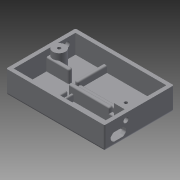
# Autodesk Inventor part: box
Saved by Autodesk Inventor 2014 SP2 (Build 180246200, 246)
## iProperties
Created: 2024-05-21
Part Number: box
Material: Generic
Document SubType Name: Sheet Metal
Designer: GauchoHP
Density: 1 g/cm^3
Sheet Metal Rule: Default_mm
Appearance: Default
Author: GauchoHP
Autodesk Inventor part; units mm, degrees
ref_plane "YZ Plane" through (0, 0, 0) normal (1, 0, 0) x (0, 1, 0)
ref_plane "XZ Plane" through (0, 0, 0) normal (0, 1, 0) x (-1, 0, 0)
ref_plane "XY Plane" through (0, 0, 0) normal (0, 0, 1) x (1, 0, 0)
sketch "Sketch1" plane through (0, 0, 0) normal (0, 0, 1) x (1, 0, 0)
  line L0 (-39, 17.5) -> (39, 17.5)
  line L1 (39, 17.5) -> (39, -37.5)
  line L2 (39, -37.5) -> (-39, -37.5)
  line L3 (-39, -37.5) -> (-39, 17.5)
  point P0 (0, 0)
  dimension "d0" = 78
  dimension "d1" = 55
  dimension "d2" = 17.5
  dimension "d3" = 39
  constraints: 8 end point, 2 parallel, 1 horizontal, 1 perpendicular
  measures "d0" distance of L0.start L0.end
  measures "d1" distance of L2.end L0.start
  measures "d2" distance from line of point (0, 0) L0
  measures "d3" distance from line of point (0, 0) L3
extrude "Extrusion1" add sketch "Sketch1" along normal blind 3
sketch "Sketch2" plane through (0, 0, 3) normal (0, 0, 1) x (1, 0, 0)
  line L0 (39, 17.5) -> (-39, 17.5) projected
  line L1 (-39, 17.5) -> (-39, -37.5) projected
  line L2 (-39, -37.5) -> (39, -37.5) projected
  line L3 (39, -37.5) -> (39, 17.5) projected
  line L4 (-36, 14.5) -> (36, 14.5)
  line L5 (36, 14.5) -> (36, -34.5)
  line L6 (36, -34.5) -> (-36, -34.5)
  line L7 (-36, -34.5) -> (-36, 14.5)
  point P0 (0, 0)
  dimension "d6" = 3
  constraints: 8 end point, 3 other
  measures "d6" distance between parallel lines of L1 L7
extrude "Extrusion2" add sketch "Sketch2" along normal blind 15
sketch "Sketch3" plane through (0, 0, 3) normal (0, 0, 1) x (1, 0, 0)
  line L0 (36, -34.5) -> (36, 14.5) projected
  line L1 (-36, -34.5) -> (36, -34.5) projected
  line L2 (36, -18.5) -> (-7.5, -18.5)
  line L3 (-9, -17) -> (-9, -17)
  line L4 (-7.5, -15.5) -> (36, -15.5)
  line L5 (36, -15.5) -> (36, -18.5)
  line L6 (-36, 14.5) -> (-36, -34.5) projected
  line L7 (-36, -5.5) -> (-19.5, -5.5)
  line L8 (-18, -7) -> (-18, -7)
  line L9 (-19.5, -8.5) -> (-36, -8.5)
  line L10 (-36, -8.5) -> (-36, -5.5)
  arc A0 (-19.5, -8.5) -> (-18, -7) centre (-19.5, -7) ccw
  arc A1 (-18, -7) -> (-19.5, -5.5) centre (-19.5, -7) ccw
  arc A2 (-7.5, -15.5) -> (-9, -17) centre (-7.5, -17) ccw
  arc A3 (-9, -17) -> (-7.5, -18.5) centre (-7.5, -17) ccw
  point P0 (0, 0)
  point P1 (-9, -15.5)
  point P2 (-9, -18.5)
  point P3 (-18, -8.5)
  point P4 (-18, -5.5)
  dimension "d9" = 3
  dimension "d10" = 45
  dimension "d11" = 16
  dimension "d17" = 18
  dimension "d18" = 3
  dimension "d19" = 26
  dimension "d57" = 1.5
  constraints: 16 end point, 10 point on line, 8 point on circle, 8 tangent, 4 centre point, 4 parallel, 3 equal radius, 2 horizontal, 2 perpendicular
  measures "d9" distance of point (-9, -18.5) point (-9, -15.5)
  measures "d10" distance of point (-9, -15.5) L4.end
  measures "d11" distance between parallel lines of L1 L2
  measures "d17" distance of point (-18, -8.5) L9.end
  measures "d18" distance of point (-18, -5.5) point (-18, -8.5)
  measures "d19" distance between parallel lines of L1 L9
  measures "d57" radius of A0
extrude "Extrusion3" add sketch "Sketch3" along normal blind 10
sketch "Sketch4" plane through (0, 0, 13) normal (0, 0, 1) x (1, 0, 0)
  line L0 (36, -15.5) -> (-7.5, -15.5) projected
  line L1 (-7.5, -18.5) -> (36, -18.5) projected
  line L2 (23.9349, -15.5) -> (26.9349, -15.5)
  line L3 (26.9349, -15.5) -> (26.9349, -18.5)
  line L4 (26.9349, -18.5) -> (23.9349, -18.5)
  line L5 (23.9349, -18.5) -> (23.9349, -15.5)
  point P0 (-9, -15.5)
  point P1 (-9, -18.5)
  point P2 (0, 0)
  dimension "d14" = 3
  constraints: 8 end point, 2 parallel, 2 point on line, 1 horizontal, 1 perpendicular
  measures "d14" distance of L2.start L2.end
extrude "Extrusion4" cut sketch "Sketch4" against normal blind 4
sketch "Sketch5" plane through (36, -34.5, 18) normal (-1, 0, 0) x (0, 0, 1)
  circle A0 centre (-5, 14) radius 2
  line L0 (-15, 0) -> (0, 0) projected
  line L1 (-15, 0) -> (-15, 16) projected
  line L2 (-15, 2) -> (-8.5, 2)
  line L3 (-8.5, 2) -> (-8.5, 14)
  line L4 (-8.5, 14) -> (-15, 14)
  line L5 (-15, 14) -> (-15, 2)
  line L6 (0, 49) -> (0, 0) projected
  line L7 (-5, 16) -> (-15, 16) projected
  point P0 (-18, 34.5)
  dimension "d20" = 4
  dimension "d38" = 14
  dimension "d39" = 12
  dimension "d40" = 2
  dimension "d41" = 6.5
  dimension "d42" = 0
  dimension "d62" = 5
  dimension "d94" = 16
  constraints: 8 end point, 2 parallel, 1 centre point, 1 horizontal, 1 perpendicular
  measures "d20" diameter of A0
  measures "d38" distance from line of L0 A0.centre
  measures "d39" distance of L2.end L3.end
  measures "d40" distance between parallel lines of L0 L2
  measures "d41" distance of L3.end L4.end
  measures "d42" distance between parallel lines of L1 L5
  measures "d62" distance from line of L6 A0.centre
  measures "d94" distance between parallel lines of L0 L7
extrude "Extrusion5" cut sketch "Sketch5" against normal blind 4
sketch "Sketch6" plane through (0, 0, 3) normal (0, 0, 1) x (1, 0, 0)
  line L0 (36, 14.5) -> (-36, 14.5) projected
  line L1 (-14, 14.5) -> (-11, 14.5)
  line L2 (-11, 14.5) -> (-11, -7)
  line L3 (-12.5, -8.5) -> (-12.5, -8.5)
  line L4 (-14, -7) -> (-14, 14.5)
  line L5 (36, -15.5) -> (36, 14.5) projected
  line L6 (-7.5, -15.5) -> (36, -15.5) projected
  line L7 (24.5, -11.5) -> (-7.5, -11.5)
  line L8 (-9, -10) -> (-9, -10)
  line L9 (-7.5, -8.5) -> (24.5, -8.5)
  line L10 (26, -10) -> (26, -10)
  arc A0 (26, -10) -> (24.5, -8.5) centre (24.5, -10) ccw
  arc A1 (24.5, -11.5) -> (26, -10) centre (24.5, -10) ccw
  arc A2 (-9, -10) -> (-7.5, -11.5) centre (-7.5, -10) ccw
  arc A3 (-7.5, -8.5) -> (-9, -10) centre (-7.5, -10) ccw
  arc A4 (-12.5, -8.5) -> (-11, -7) centre (-12.5, -7) ccw
  arc A5 (-14, -7) -> (-12.5, -8.5) centre (-12.5, -7) ccw
  point P0 (0, 0)
  point P1 (-11, -8.5)
  point P2 (-14, -8.5)
  point P3 (-9, -15.5)
  point P4 (26, -11.5)
  point P5 (-9, -8.5)
  point P6 (-9, -11.5)
  point P7 (26, -8.5)
  dimension "d23" = 3
  dimension "d24" = 23
  dimension "d25" = 0
  dimension "d33" = 47
  dimension "d35" = 3
  dimension "d36" = 4
  dimension "d37" = 23
  dimension "d54" = 35
  dimension "d55" = 10
  dimension "d56" = 1.5
  constraints: 16 end point, 12 point on circle, 12 point on line, 12 tangent, 6 centre point, 5 equal radius, 4 parallel, 2 horizontal, 2 perpendicular
  measures "d23" distance of point (-11, -8.5) point (-14, -8.5)
  measures "d24" distance of L1.end point (-11, -8.5)
  measures "d25" distance between parallel lines of L0 L1
  measures "d33" distance between parallel lines of L2 L5
  measures "d35" distance of point (-9, -11.5) point (-9, -8.5)
  measures "d36" distance between parallel lines of L7 L6
  measures "d37" distance between parallel lines of L0 L9
  measures "d54" distance between parallel lines of L10 L8
  measures "d55" distance between parallel lines of L5 L10
  measures "d56" radius of A0
extrude "Extrusion6" add sketch "Sketch6" along normal blind 5
chamfer "Chamfer1" distance 2 angle 45 4 edges at (37.5, -20.5, 3) (37.5, -32.5, 3) (37.5, -32.5, 9.5) (37.5, -20.5, 9.5)
sketch "Sketch8" plane through (0, 0, 3) normal (0, 0, 1) x (1, 0, 0)
  circle A0 centre (32, -13.5) radius 5
  line L0 (39, 17.5) -> (39, -37.5) projected
  circle A1 centre (32, -13.5) radius 1.25
  line L1 (36, -34.5) -> (36, 14.5) projected
  line L2 (-36, 14.5) -> (-36, -5.5) projected
  line L3 (-36, -5.5) -> (-19.5, -5.5) projected
  circle A2 centre (-32, -2.5) radius 5
  line L4 (-39, -37.5) -> (-39, 17.5) projected
  line L5 (39, 17.5) -> (-39, 17.5) projected
  circle A3 centre (-32, -2.5) radius 1.25
  point P0 (0, 0)
  point P1 (36, -8.5)
  dimension "d46" = 10
  dimension "d47" = 7
  dimension "d50" = 2.5
  dimension "d51" = 4
  dimension "d63" = 10
  dimension "d64" = 3
  dimension "d65" = 4
  dimension "d66" = 7
  dimension "d67" = 20
  dimension "d68" = 31
  dimension "d69" = 2.5
  constraints: 4 centre point, 2 coincident
  measures "d46" diameter of A0
  measures "d47" distance from line of L0 A0.centre
  measures "d50" diameter of A1
  measures "d51" distance from line of L1 A1.centre
  measures "d63" diameter of A2
  measures "d64" distance from line of L3 A2.centre
  measures "d65" distance from line of L2 A2.centre
  measures "d66" distance from line of L4 A2.centre
  measures "d67" distance from line of A2.centre L5
  measures "d68" distance from line of L5 A0.centre
  measures "d69" diameter of A3
extrude "Extrusion7" add sketch "Sketch8" along normal blind 15
sketch "Sketch10" plane through (-36, -34.5, 18) normal (1, 0, 0) x (0, 0, -1)
  circle A0 centre (5, 42) radius 2.5
  line L0 (0, 0) -> (0, 49) projected
  line L1 (15, 49) -> (0, 49) projected
  point P0 (18, 34.5)
  dimension "d58" = 5
  dimension "d61" = 5
  dimension "d71" = 7
  constraints: 1 centre point
  measures "d58" diameter of A0
  measures "d61" distance from line of L0 A0.centre
  measures "d71" distance from line of L1 A0.centre
extrude "Extrusion9" cut sketch "Sketch10" against normal blind 3
fillet "Fillet1" radius 1 4 edges at (39, -37.5, 9) (39, 17.5, 9) (-39, 17.5, 9) (-39, -37.5, 9)
sketch "Sketch11" plane through (0, 0, 13) normal (0, 0, 1) x (1, 0, 0)
  arc A0 (32, -18.5) -> (36, -16.5) centre (32, -13.5) ccw projected
  line L0 (32, -18.5) -> (36, -18.5) projected
  line L1 (36, -16.5) -> (36, -18.5) projected
  point P0 (0, 0)
extrude "Extrusion10" add sketch "Sketch11" along normal blind 5
sketch "Sketch12" plane through (0, 0, 13) normal (0, 0, 1) x (1, 0, 0)
  arc A0 (27.4174, -15.5) -> (32, -18.5) centre (32, -13.5) ccw projected
  line L0 (27.4174, -15.5) -> (26.9349, -15.5) projected
  line L1 (26.9349, -15.5) -> (26.9349, -18.5) projected
  line L2 (26.9349, -18.5) -> (32, -18.5) projected
  point P0 (0, 0)
extrude "Extrusion11" add sketch "Sketch12" along normal blind 5
fillet "Fillet2" radius 1 5 edges at (26.9349, -15.5, 13.5) (25.4349, -15.5, 9) (23.9349, -15.5, 11) (26.9349, -18.5, 13.5) (23.9349, -18.5, 11)
fillet "Fillet3" radius 1 10 edges at (7.7174, -18.5, 13) (23.642, -18.2071, 13) (23.9349, -17, 13) (23.642, -15.7929, 13) (7.7174, -15.5, 13) (-9, -17, 13) (25.4349, -18.5, 9) (-18, -7, 13) (-23.75, -5.5, 13) (-27.75, -8.5, 13)
fillet "Fillet4" radius 1 7 edges at (26, -10, 8) (8.5, -8.5, 8) (-9, -10, 8) (8.5, -11.5, 8) (-12.5, -8.5, 8) (-11, 3.75, 8) (-14, 3.75, 8)
sketch "Sketch13" plane through (0, 0, 3) normal (0, 0, 1) x (1, 0, 0)
  line L0 (-36, -34.5) -> (36, -34.5) projected
  line L1 (-11, -18.5) -> (-9, -18.5)
  line L2 (-9, -18.5) -> (-9, -34.5)
  line L3 (-9, -34.5) -> (-11, -34.5)
  line L4 (-11, -34.5) -> (-11, -18.5)
  line L5 (36, -22.5) -> (36, -18.5) projected
  line L6 (36, -18.5) -> (-7.5, -18.5) projected
  line L7 (-6.5, -34.5) -> (-4.5, -34.5)
  line L8 (-4.5, -34.5) -> (-4.5, -18.5)
  line L9 (-4.5, -18.5) -> (-6.5, -18.5)
  line L10 (-6.5, -18.5) -> (-6.5, -34.5)
  point P0 (0, 0)
  dimension "d79" = 2
  dimension "d80" = 16
  dimension "d91" = 45
  dimension "d92" = 2
  dimension "d93" = 40.5
  constraints: 16 end point, 4 parallel, 3 point on line, 2 horizontal, 2 perpendicular
  measures "d79" distance of L2.end L3.end
  measures "d80" distance of L3.end L1.start
  measures "d91" distance between parallel lines of L2 L5
  measures "d92" distance of L7.start L7.end
  measures "d93" distance between parallel lines of L5 L8
extrude "Extrusion12" add sketch "Sketch13" along normal blind 5
fillet "Fillet5" radius 0.9 7 edges at (-10, -18.5, 8) (-11, -26.5, 8) (-9, -26.5, 8) (-9, -18.5, 5.5) (-11, -18.5, 5.5) (-6.5, -26.5, 8) (-4.5, -26.5, 8)
chamfer "Chamfer2" distance 1 angle 45 8 edges at (0, -37.5, 0) (-38.7071, -37.2071, 0) (-39, -10, 0) (-38.7071, 17.2071, 0) (0, 17.5, 0) (38.7071, 17.2071, 0) (39, -10, 0) (38.7071, -37.2071, 0)
fillet "Fillet6" radius 2 8 edges at (-38.7071, -37.2071, 1) (-39, -10, 1) (-38.7071, 17.2071, 1) (0, 17.5, 1) (38.7071, 17.2071, 1) (39, -10, 1) (38.7071, -37.2071, 1) (0, -37.5, 1)
fillet "Fillet7" radius 2 4 edges at (37.5, -20.5, 5) (37.5, -32.5, 5) (37.5, -30.5, 3) (37.5, -22.5, 3)
equation "\"BendRadius\" = Thickness"
equation "\"BendReliefWidth\" = Thickness"
equation "\"BendReliefDepth\" = 0.5 * Thickness"
equation "\"CornerReliefSize\" = 4 * Thickness"
equation "\"MinimumRemnant\" = 2 * Thickness"
equation "\"TransitionRadius\" = BendRadius"
equation "\"JacobiRadiusSize\" = BendRadius"
equation "\"GapSize\" = Thickness"
equation "\"Thickness\" = 0.5"
body "Solid1"
